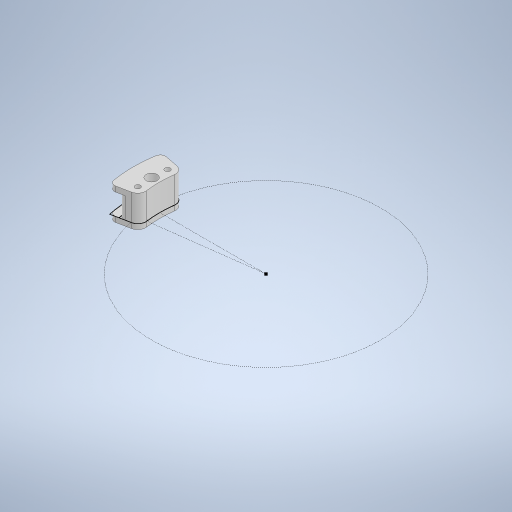
# Autodesk Inventor part: Braces
Saved by Autodesk Inventor 2023.2 (Build 272271000, 271)
## iProperties
Created: 2023-04-12
Part Number: Braces
Material: Generic
Document SubType Name: Modeling
Designer: Nathan Cai
Density: 1 g/cm^3
Appearance: Default
Mass: 4.90637 g
Surface Area: 30.5635 cm^2
Volume: 4.90637 cm^3
Author: Nathan Cai
Autodesk Inventor part; units mm, degrees
ref_plane "YZ Plane" through (0, 0, 0) normal (1, 0, 0) x (0, 1, 0)
ref_plane "XZ Plane" through (0, 0, 0) normal (0, 1, 0) x (-1, 0, 0)
sketch "Sketch1" plane through (0, 0, 0) normal (0, 1, 0) x (-1, 0, 0)
  circle A0 centre (0, 0) radius 3.302
  line L0 (0, 0) -> (3.302, 0)
  arc A1 (6.35, 0) -> (4.8481, 14.975) centre (-69.0563, 0) ccw
  circle A2 centre (-69.0563, 0) radius 69.0563 construction
  circle A3 centre (-0.5908, 9.0136) radius 1.5875
  line L1 (-0.5908, 9.0136) -> (-69.0563, 0) construction
  circle A4 centre (-0.5908, 9.0136) radius 4.7625
  line L2 (9.5157, 15.9208) -> (-1.5366, 13.6813)
  arc A5 (11.1125, 0) -> (9.5157, 15.9208) centre (-69.0563, 0) ccw
  arc A6 (-4.7625, 0) -> (-5.3125, 8.392) centre (-69.0563, 0) ccw
  line L3 (0, 0) -> (-69.0563, 0) construction
  arc A7 (4.8481, -14.975) -> (6.35, 0) centre (-69.0563, 0) ccw
  circle A8 centre (-0.5908, -9.0136) radius 1.5875
  circle A9 centre (-0.5908, -9.0136) radius 4.7625
  line L4 (9.5157, -15.9208) -> (-1.5366, -13.6813)
  arc A10 (9.5157, -15.9208) -> (11.1125, 0) centre (-69.0563, 0) ccw
  arc A11 (-5.3125, -8.392) -> (-4.7625, 0) centre (-69.0563, 0) ccw
  point P0 (4.8277, -15.4708)
  dimension "d0" = 6.604
  dimension "d1" = 6.35
  dimension "d2" = 75.4062
  dimension "d3" = 3.175
  dimension "d6" = 9.525
  dimension "d7" = 4.7625
  dimension "d8" = 7.5
  dimension "d14" = 138.1125
  constraints: 18 point on circle, 11 centre point, 10 end point, 6 symmetric about line, 5 point on line, 4 coincident, 2 concentric, 2 horizontal, 2 tangent, 1 horizontal alignment, 1 line through centre, 7 other
  measures "d1" distance of A1.start point (0, 0)
  measures "d2" radius of A1
  measures "d3" diameter of A3
  measures "d6" diameter of A4
  measures "d7" radial gap between concentric circles of A1 A5
  measures "d8" angle of L3 L1
  measures "d14" diameter of A2
extrude "Extrusion1" add sketch "Sketch1" along normal blind 12.7 contours A7 L4 A9 A11 A6 A4 L2 A1 | A4 | A9
extrude "Extrusion2" add sketch "Sketch1" against normal blind 3.175
ref_plane "Work Plane1" through (0, 6.35, 0) normal (0, 1, 0) x (1, 0, 0)
mirror "Mirror1" about plane through (0, 6.35, 0) normal (0, 1, 0) of "Extrusion2"
fillet "Fillet1" radius 3.175 6 edges at (-9.5157, 14.2875, 15.9208) (-9.5157, 14.2875, -15.9208) (-9.5157, -1.5875, -15.9208) (-9.5157, -1.5875, 15.9208) (-4.8481, 6.35, 14.975) (-4.8481, 6.35, -14.975)
body "Solid1"
